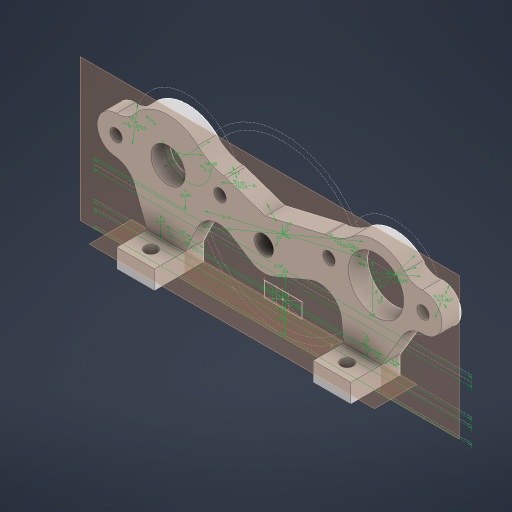
# Autodesk Inventor part: Motormount
Saved by Autodesk Inventor 2023.5 (Build 275446000, 446)
## iProperties
Created: 2024-12-07
Part Number: Motormount
Material: 一般
Document SubType Name: Modeling
Designer: IshiiLabHonda
Density: 1 g/cm^3
Appearance: 既定
Author: IshiiLabHonda
Autodesk Inventor part; units mm, degrees
ref_plane "YZ Plane" through (0, 0, 0) normal (1, 0, 0) x (0, 1, 0)
ref_plane "XZ Plane" through (0, 0, 0) normal (0, 1, 0) x (-1, 0, 0)
ref_plane "XY Plane" through (0, 0, 0) normal (0, 0, 1) x (1, 0, 0)
sketch "blueprint" plane through (0, 0, 0) normal (0, 0, 1) x (1, 0, 0)
  line L0 (0, 0) -> (0, 1) construction
  line L1 (0, 0) -> (1, 0) construction
  circle A0 centre (0, 0) radius 1.25
  circle A1 centre (0, 0) radius 11.5 construction
  line L2 (-25, -11.5) -> (25, -11.5) construction
  line L3 (-25, -9.5) -> (25, -9.5) construction
  line L4 (-25, -8.5) -> (25, -8.5) construction
  line L5 (-25, -4.5) -> (25, -4.5) construction
  circle A2 centre (0, 0) radius 10.65 construction
  circle A3 centre (-12.6949, 2.8) radius 2.25
  circle A4 centre (14.8381, 2.8) radius 4.35 construction
  circle A5 centre (14.8381, 2.8) radius 3.6 construction
  line L6 (-25, -3.7) -> (25, -3.7) construction
  circle A6 centre (-12.6949, 2.8) radius 4.26 construction
  circle A7 centre (-19.5799, 2.8) radius 0.625 construction
  circle A8 centre (-5.8099, 2.8) radius 0.625 construction
  circle A9 centre (-12.6949, 2.8) radius 6.885 construction
  circle A10 centre (-19.5799, 2.8) radius 1.825
  circle A11 centre (-5.8099, 2.8) radius 1.825
  circle A12 centre (14.8381, 2.8) radius 5.1
  circle A13 centre (14.8381, 2.8) radius 6.225 construction
  circle A14 centre (21.0631, 2.8) radius 0.625 construction
  circle A15 centre (8.6131, 2.8) radius 0.625 construction
  circle A16 centre (21.0631, 2.8) radius 1.825
  circle A17 centre (-19.5799, 2.8) radius 0.8
  circle A18 centre (-5.8099, 2.8) radius 0.8
  circle A19 centre (21.0631, 2.8) radius 0.8
  circle A20 centre (-19.5799, 2.8) radius 2.5
  circle A21 centre (-5.8099, 2.8) radius 2.5
  circle A22 centre (21.0631, 2.8) radius 2.5
  circle A23 centre (14.8381, 2.8) radius 3.65
  circle A24 centre (0, 0) radius 3.25
  line L7 (-15, -4.5) -> (-15, -8.5) construction
  line L8 (15, -4.5) -> (15, -8.5) construction
  line L9 (-10.5, -8.5) -> (-10.5, -6)
  line L10 (-15.5, -8.5) -> (-15.5, -6)
  line L11 (-15.5, -6) -> (-10.5, -6)
  line L12 (-13, -6) -> (-13, -8.5)
  line L13 (-13.8, -6) -> (-13.8, -8.5)
  line L14 (-12.2, -6) -> (-12.2, -8.5)
  line L15 (10.5, -8.5) -> (10.5, -6)
  line L16 (15.5, -8.5) -> (15.5, -6)
  line L17 (15.5, -6) -> (10.5, -6)
  line L18 (13, -6) -> (13, -8.5)
  line L19 (13.8, -6) -> (13.8, -8.5)
  line L20 (12.2, -6) -> (12.2, -8.5)
  line L21 (-15.5, -8.5) -> (-10.5, -8.5)
  line L22 (10.5, -8.5) -> (15.5, -8.5)
  circle A25 centre (8.6131, 2.8) radius 1.825
  line L23 (-12.6949, 2.8) -> (-19.5799, 2.8) construction
  line L24 (-12.6949, 2.8) -> (-5.8099, 2.8) construction
  line L25 (14.8381, 2.8) -> (8.6131, 2.8) construction
  circle A26 centre (-12.6949, 2.8) radius 5.76
  line L26 (-2.5, -6.5) -> (2.5, -6.5)
  line L27 (2.5, -6.5) -> (2.5, -8.5)
  line L28 (2.5, -8.5) -> (-2.5, -8.5)
  line L29 (-2.5, -8.5) -> (-2.5, -6.5)
  line L30 (-2.5, -6.5) -> (2.5, -8.5) construction
  line L31 (2.5, -6.5) -> (-2.5, -8.5) construction
  line L32 (0, -6.5) -> (0, -8.5) construction
  line L33 (-0.8, -6.5) -> (-0.8, -8.5) construction
  line L34 (0.8, -6.5) -> (0.8, -8.5) construction
  circle A27 centre (8.6131, 2.8) radius 0.8
  circle A28 centre (8.6131, 2.8) radius 2.5
  line L35 (21.0631, 2.8) -> (14.8381, 2.8) construction
  circle A29 centre (0, 0) radius 2.15
  point P0 (19.5378, 0.8193)
  point P1 (19.5378, 4.7807)
  point P2 (0, -8.5)
  point P3 (-6.4807, -9.5)
  point P4 (6.4807, -9.5)
  point P5 (0, -7.5)
  point P6 (-18.0929, 0.7903)
  point P7 (-7.2969, 0.7903)
  point P8 (-7.2969, 4.8097)
  point P9 (-18.0929, 4.8097)
  dimension "d0" = 1
  dimension "d1" = 1
  dimension "d2" = 2.5
  dimension "d3" = 23
  dimension "d4" = 50
  dimension "d5" = 50
  dimension "d6" = 2
  dimension "d7" = 50
  dimension "d9" = 1
  dimension "d10" = 50
  dimension "d12" = 4
  dimension "d13" = 21.3
  dimension "d14" = 4.5
  dimension "d15" = 8.7
  dimension "d17" = 0.1
  dimension "d18" = 0.1
  dimension "d20" = 7.2
  dimension "d21" = 50
  dimension "d22" = 0.8
  dimension "d23" = 8.52
  dimension "d26" = 1.25
  dimension "d27" = 1.25
  dimension "d28" = 1.2
  dimension "d29" = 1.2
  dimension "d31" = 1.5
  dimension "d32" = 1.25
  dimension "d33" = 1.25
  dimension "d34" = 1.2
  dimension "d37" = 0.5
  dimension "d40" = 1.6
  dimension "d41" = 1.6
  dimension "d43" = 1.6
  dimension "d48" = 7.3
  dimension "d49" = 2
  dimension "d56" = 30
  dimension "d90" = 2.5
  dimension "d92" = 5
  dimension "d93" = 1.6
  dimension "d104" = 1.2
  dimension "d105" = 5
  dimension "d106" = 1.6
  dimension "d107" = 2.5
  dimension "d129" = 5
  dimension "d130" = 5
  dimension "d132" = 5
  dimension "d155" = 26
  dimension "d158" = 1.5
  dimension "d160" = 0.5
  dimension "d161" = 180
  dimension "d166" = 1.6
  dimension "d167" = 5
  dimension "d168" = 2
  dimension "d178" = 1.6
  dimension "d179" = 5
  dimension "d180" = 180
  dimension "d181" = 6.5
  dimension "d187" = 2.24
  dimension "d196" = 4.3
  constraints: 70 end point, 30 centre point, 25 coincident, 17 point on line, 10 parallel, 8 midpoint, 7 vertical, 6 point on circle, 5 symmetric about line, 4 perpendicular, 3 horizontal, 1 tangent, 18 other
  measures "d0" distance of L0.start L0.end
  measures "d1" distance of L0.start L1.end
  measures "d2" diameter of A0
  measures "d3" diameter of A1
  measures "d4" distance of L2.start L2.end
  measures "d5" distance of L3.start L3.end
  measures "d6" distance between parallel lines of L2 L3
  measures "d7" distance of point (-25, -8.5) point (25, -8.5)
  measures "d10" distance of L5.start L5.end
  measures "d13" diameter of A2
  measures "d14" diameter of A3
  measures "d15" diameter of A4
  measures "d20" diameter of A5
  measures "d21" distance of L6.start L6.end
  measures "d22" distance between parallel lines of L5 L6
  measures "d23" diameter of A6
  measures "d26" diameter of A8
  measures "d27" diameter of A7
  measures "d28" radial gap between concentric circles of A10 A7
  measures "d29" radial gap between concentric circles of A11 A8
  measures "d31" radial gap between concentric circles of A12 A5
  measures "d32" diameter of A14
  measures "d33" diameter of A15
  measures "d34" radial gap between concentric circles of A14 A16
  measures "d40" diameter of A17
  measures "d41" diameter of A18
  measures "d43" diameter of A19
  measures "d48" diameter of A23
  measures "d49" radial gap between concentric circles of A24 A0
  measures "d56" distance between parallel lines of L8 L7
  measures "d90" distance of L10.start L10.end
  measures "d92" distance between parallel lines of L9 L10
  measures "d93" distance between parallel lines of L14 L13
  measures "d104" radial gap between concentric circles of A25 A15
  measures "d105" distance between parallel lines of L16 L15
  measures "d106" distance between parallel lines of L19 L20
  measures "d107" distance of L15.start L15.end
  measures "d129" diameter of A20
  measures "d130" diameter of A21
  measures "d132" diameter of A22
  measures "d155" distance between parallel lines of L18 L12
  measures "d158" radial gap between concentric circles of A26 A6
  measures "d161" angle of L24 L23
  measures "d166" distance between parallel lines of L33 L34
  measures "d167" distance between parallel lines of L27 L29
  measures "d168" distance between parallel lines of L26 L28
  measures "d178" diameter of A27
  measures "d179" diameter of A28
  measures "d180" angle of L25 L35
  measures "d181" distance between parallel lines of L6 L25
  measures "d187" distance edge to line of A6 L6
  measures "d196" diameter of A29
sketch "スケッチ5" plane through (0, 0, 0) normal (0, 0, 1) x (1, 0, 0)
  circle A0 centre (0, 0) radius 10.65 construction
  circle A1 centre (0, 0) radius 11.5 construction
  line L0 (-25, -3.7) -> (25, -3.7) construction
  line L1 (-25, -4.5) -> (25, -4.5) construction
  line L2 (-25, -8.5) -> (25, -8.5) construction
  line L3 (-25, -9.5) -> (25, -9.5) construction
  line L4 (-25, -11.5) -> (25, -11.5) construction
  line L5 (0, 0) -> (1, 0) construction
  circle A2 centre (0, 0) radius 1.25 projected
  line L6 (0, 0) -> (0, 1) construction
  circle A3 centre (-5.8099, 2.8) radius 0.625 construction
  circle A4 centre (-5.8099, 2.8) radius 0.8 projected
  circle A5 centre (-5.8099, 2.8) radius 1.825 construction
  circle A6 centre (-5.8099, 2.8) radius 2.5 projected
  line L7 (-12.6949, 2.8) -> (-5.8099, 2.8) construction
  circle A7 centre (-12.6949, 2.8) radius 2.25 projected
  circle A8 centre (-12.6949, 2.8) radius 4.26 construction
  circle A9 centre (-12.6949, 2.8) radius 5.76 projected
  circle A10 centre (-12.6949, 2.8) radius 6.885 construction
  line L8 (-12.6949, 2.8) -> (-19.5799, 2.8) construction
  circle A11 centre (-19.5799, 2.8) radius 2.5 projected
  circle A12 centre (14.8381, 2.8) radius 3.6 construction
  circle A13 centre (14.8381, 2.8) radius 4.35 construction
  circle A14 centre (-19.5799, 2.8) radius 0.625 construction
  circle A15 centre (-19.5799, 2.8) radius 0.8 projected
  circle A16 centre (-19.5799, 2.8) radius 1.825 construction
  circle A17 centre (14.8381, 2.8) radius 5.1 projected
  circle A18 centre (14.8381, 2.8) radius 6.225 construction
  circle A19 centre (21.0631, 2.8) radius 0.625 construction
  circle A20 centre (8.6131, 2.8) radius 0.625 construction
  circle A21 centre (21.0631, 2.8) radius 1.825 construction
  line L9 (14.8381, 2.8) -> (8.6131, 2.8) construction
  circle A22 centre (8.6131, 2.8) radius 0.8 projected
  circle A23 centre (8.6131, 2.8) radius 1.825 construction
  circle A24 centre (8.6131, 2.8) radius 2.5 projected
  circle A25 centre (14.8381, 2.8) radius 3.65 projected
  line L10 (21.0631, 2.8) -> (14.8381, 2.8) construction
  circle A26 centre (21.0631, 2.8) radius 2.5 projected
  circle A27 centre (21.0631, 2.8) radius 0.8 projected
  line L11 (-10.5, -8.5) -> (-10.5, -6) projected
  line L12 (-12.2, -6) -> (-12.2, -8.5) projected
  line L13 (-15.5, -6) -> (-10.5, -6) projected
  line L14 (-13, -6) -> (-13, -8.5) projected
  line L15 (-13.8, -6) -> (-13.8, -8.5) projected
  line L16 (-15.5, -8.5) -> (-10.5, -8.5) projected
  line L17 (-15, -4.5) -> (-15, -8.5) construction
  line L18 (-15.5, -8.5) -> (-15.5, -6) projected
  line L19 (15, -4.5) -> (15, -8.5) construction
  line L20 (15.5, -8.5) -> (15.5, -6) projected
  line L21 (13.8, -6) -> (13.8, -8.5) projected
  line L22 (15.5, -6) -> (10.5, -6) projected
  line L23 (13, -6) -> (13, -8.5) projected
  line L24 (12.2, -6) -> (12.2, -8.5) projected
  line L25 (10.5, -8.5) -> (15.5, -8.5) projected
  line L26 (10.5, -8.5) -> (10.5, -6) projected
  circle A28 centre (0, 0) radius 3.25 projected
  line L27 (-2.5, -8.5) -> (-2.5, -6.5) projected
  line L28 (-0.8, -6.5) -> (-0.8, -8.5) construction
  line L29 (0, -6.5) -> (0, -8.5) construction
  line L30 (0.8, -6.5) -> (0.8, -8.5) construction
  line L31 (-2.5, -6.5) -> (2.5, -6.5) projected
  line L32 (-2.5, -6.5) -> (2.5, -8.5) construction
  line L33 (2.5, -6.5) -> (-2.5, -8.5) construction
  line L34 (2.5, -8.5) -> (-2.5, -8.5) projected
  line L35 (2.5, -6.5) -> (2.5, -8.5) projected
  line L36 (-15.5, -6) -> (-18.0759, 0.7451)
  line L37 (-10.5, -6) -> (-7.4926, 0.3274)
  line L38 (10.5, -6) -> (9.7581, 2.3486)
  line L39 (15.5, -6) -> (19.2096, 0.1731)
  line L40 (-7.1498, 0.6894) -> (-1.7419, -2.7438)
  line L41 (-4.9938, 5.163) -> (1.0609, 3.072)
  line L42 (-0.7454, 3.1634) -> (8.0398, 5.2334)
  line L43 (1.2573, -2.997) -> (9.5803, 0.4946)
  point P0 (0, -7.5)
  point P1 (0, -8.5)
  point P2 (6.4807, -9.5)
  point P3 (-6.4807, -9.5)
  point P4 (10.1385, 0.8193)
  point P5 (9.9081, 0.6615)
  point P6 (0.171, 3.3793)
  point P7 (-18.0929, 4.8097)
  point P8 (-18.0929, 0.7903)
  point P9 (-7.2969, 0.7903)
  point P10 (19.5378, 0.8193)
  point P11 (19.5378, 4.7807)
  point P12 (10.1385, 4.7807)
  point P13 (-7.2969, 4.8097)
  constraints: 16 end point, 12 point on circle, 12 tangent, 5 other
extrude "押し出し33" add sketch "スケッチ5" along normal blind 2.5 contours A6 A9 | A6 L41 L42 A28 L40 | A9 A6 | A6 A9 A11 | L42 A24 L43 A28 L41 | L41 A28 L42 | A28 | A11 A9 | A9 A11 | A24 A17 L38 | L37 L13 L36 A9 | A24 A17 | A17 A26 A24 | L11 L16 L12 L13 | L38 A17 A24 | A24 A17 L39 L22 L38 | A26 A17 | A17 A26 | L13 L15 L16 L18 | L12 L16 L14 L13 | L22 L24 L25 L26 | L13 L14 L16 L15 | L22 L23 L25 L24 | L20 L25 L21 L22 | L22 L21 L25 L23
extrude "押し出し34" cut sketch "blueprint" along normal blind 0.5 contours A10 A26 | A26 A10 | A26 A11 | A11 A26 | A12 A16 | A12 A16 | A25 A12 | A12 A25 | A17 | A19 | A29
fillet "フィレット2" radius 7 2 edges at (10.1385, 4.7807, 1.25) (-7.2969, 4.8097, 1.25)
fillet "フィレット3" radius 3 6 edges at (9.9081, 0.6615, 1.25) (-7.2969, 0.7903, 1.25) (-18.0929, 0.7903, 1.25) (-18.0929, 4.8097, 1.25) (19.5378, 4.7807, 1.25) (19.5378, 0.8193, 1.25)
ref_plane "作業平面6" through (0, 0, 2.5) normal (0, 0, 1) x (1, 0, 0)
sketch "スケッチ7" plane through (0, 0, 2.5) normal (0, 0, 1) x (1, 0, 0)
  line L0 (-4.4189, -1.0443) -> (-1.7419, -2.7438) projected
  line L1 (-10.5, -8.5) -> (-10.5, -6) projected
  line L2 (-10.5, -8.5) -> (-10.5, -6) projected
  line L3 (-4.4189, -1.0443) -> (-1.7419, -2.7438) projected
  line L4 (10.5, -6) -> (10.5, -8.5) projected
  line L5 (10.5, -6) -> (10.5, -8.5) projected
  arc A0 (21.0269, 0.3003) -> (20.9393, 5.2969) centre (21.0631, 2.8) ccw projected
  arc A1 (21.0269, 0.3003) -> (20.9393, 5.2969) centre (21.0631, 2.8) ccw projected
  line L6 (10.5, -8.5) -> (15.5, -8.5) projected
  line L7 (15.5, -8.5) -> (15.5, -6) projected
  line L8 (15.5, -8.5) -> (15.5, -6) projected
  line L9 (10.5, -8.5) -> (15.5, -8.5) projected
  line L10 (-15.5, -6) -> (-15.5, -8.5) projected
  line L11 (-15.5, -6) -> (-15.5, -8.5) projected
  line L12 (-15.5, -8.5) -> (-10.5, -8.5) projected
  line L13 (-15.5, -8.5) -> (-10.5, -8.5) projected
  arc A2 (-4.4189, -1.0443) -> (-8.7363, -2.2892) centre (-6.0267, -3.577) ccw projected
  arc A3 (-1.7419, -2.7438) -> (1.2573, -2.997) centre (0, 0) ccw projected
  arc A4 (-1.7419, -2.7438) -> (1.2573, -2.997) centre (0, 0) ccw projected
  circle A5 centre (-5.8099, 2.8) radius 0.8 projected
  circle A6 centre (-5.8099, 2.8) radius 0.8 projected
  circle A7 centre (0, 0) radius 1.25 projected
  circle A8 centre (-5.8099, 2.8) radius 1.825 projected
  circle A9 centre (-5.8099, 2.8) radius 1.825 projected
  arc A10 (-4.9938, 5.163) -> (-5.329, 5.2533) centre (-5.8099, 2.8) ccw projected
  circle A11 centre (0, 0) radius 2.15 projected
  circle A12 centre (0, 0) radius 2.15 projected
  line L14 (0.171, 3.3793) -> (-4.9938, 5.163) projected
  line L15 (0.171, 3.3793) -> (-4.9938, 5.163) projected
  arc A13 (-8.762, 7.0083) -> (-5.329, 5.2533) centre (-3.9824, 12.1226) ccw projected
  arc A14 (-8.762, 7.0083) -> (-5.329, 5.2533) centre (-3.9824, 12.1226) ccw projected
  line L16 (10.2739, -3.4557) -> (10.5, -6) projected
  line L17 (10.2739, -3.4557) -> (10.5, -6) projected
  line L18 (8.0398, 5.2334) -> (0.171, 3.3793) projected
  line L19 (8.0398, 5.2334) -> (0.171, 3.3793) projected
  arc A15 (8.2451, 5.2728) -> (8.0398, 5.2334) centre (8.6131, 2.8) ccw projected
  arc A16 (8.2451, 5.2728) -> (8.0398, 5.2334) centre (8.6131, 2.8) ccw projected
  circle A17 centre (8.6131, 2.8) radius 0.8 projected
  circle A18 centre (8.6131, 2.8) radius 0.8 projected
  circle A19 centre (8.6131, 2.8) radius 1.825 projected
  circle A20 centre (8.6131, 2.8) radius 1.825 projected
  circle A21 centre (14.8381, 2.8) radius 3.65 projected
  circle A22 centre (14.8381, 2.8) radius 3.65 projected
  circle A23 centre (21.0631, 2.8) radius 0.8 projected
  circle A24 centre (0, 0) radius 1.25 projected
  arc A25 (8.2451, 5.2728) -> (11.625, 6.7605) centre (7.2148, 12.1965) ccw projected
  circle A26 centre (-12.6949, 2.8) radius 2.25 projected
  circle A27 centre (-12.6949, 2.8) radius 2.25 projected
  circle A28 centre (-19.5799, 2.8) radius 0.8 projected
  arc A29 (-8.762, 7.0083) -> (-17.1783, 6.4162) centre (-12.6949, 2.8) ccw projected
  arc A30 (-8.762, 7.0083) -> (-17.1783, 6.4162) centre (-12.6949, 2.8) ccw projected
  line L20 (-17.1744, -1.6154) -> (-15.5, -6) projected
  circle A31 centre (-19.5799, 2.8) radius 0.8 projected
  circle A32 centre (-19.5799, 2.8) radius 1.825 projected
  circle A33 centre (-19.5799, 2.8) radius 1.825 projected
  circle A34 centre (21.0631, 2.8) radius 0.8 projected
  circle A35 centre (21.0631, 2.8) radius 1.825 projected
  circle A36 centre (21.0631, 2.8) radius 1.825 projected
  arc A37 (-4.9938, 5.163) -> (-5.329, 5.2533) centre (-5.8099, 2.8) ccw projected
  line L21 (-17.1744, -1.6154) -> (-15.5, -6) projected
  arc A38 (-4.4189, -1.0443) -> (-8.7363, -2.2892) centre (-6.0267, -3.577) ccw projected
  line L22 (-10.5, -6) -> (-8.7363, -2.2892) projected
  line L23 (-10.5, -6) -> (-8.7363, -2.2892) projected
  arc A39 (8.2451, 5.2728) -> (11.625, 6.7605) centre (7.2148, 12.1965) ccw projected
  line L24 (1.2573, -2.997) -> (6.1251, -0.9548) projected
  line L25 (1.2573, -2.997) -> (6.1251, -0.9548) projected
  arc A40 (10.2739, -3.4557) -> (6.1251, -0.9548) centre (7.2857, -3.7213) ccw projected
  arc A41 (18.5861, 6.2587) -> (11.625, 6.7605) centre (14.8381, 2.8) ccw projected
  arc A42 (18.5861, 6.2587) -> (11.625, 6.7605) centre (14.8381, 2.8) ccw projected
  line L26 (15.5, -6) -> (18.412, -1.1542) projected
  line L27 (15.5, -6) -> (18.412, -1.1542) projected
  arc A43 (10.2739, -3.4557) -> (6.1251, -0.9548) centre (7.2857, -3.7213) ccw projected
  arc A44 (-17.1744, -1.6154) -> (-19.7604, 0.3065) centre (-19.977, -2.6856) ccw projected
  arc A45 (-17.1744, -1.6154) -> (-19.7604, 0.3065) centre (-19.977, -2.6856) ccw projected
  arc A46 (-19.5497, 5.2998) -> (-19.7604, 0.3065) centre (-19.5799, 2.8) ccw projected
  arc A47 (-19.5497, 5.2998) -> (-17.1783, 6.4162) centre (-19.5134, 8.2996) ccw projected
  arc A48 (-19.5497, 5.2998) -> (-19.7604, 0.3065) centre (-19.5799, 2.8) ccw projected
  arc A49 (-19.5497, 5.2998) -> (-17.1783, 6.4162) centre (-19.5134, 8.2996) ccw projected
  arc A50 (21.0269, 0.3003) -> (18.412, -1.1542) centre (20.9834, -2.6994) ccw projected
  arc A51 (21.0269, 0.3003) -> (18.412, -1.1542) centre (20.9834, -2.6994) ccw projected
  arc A52 (18.5861, 6.2587) -> (20.9393, 5.2969) centre (20.7908, 8.2933) ccw projected
  arc A53 (18.5861, 6.2587) -> (20.9393, 5.2969) centre (20.7908, 8.2933) ccw projected
  line L28 (-25, -3.7) -> (25, -3.7) construction
  line L29 (-25, -4.5) -> (25, -4.5) construction
  line L30 (-25, -8.5) -> (25, -8.5) construction
  line L31 (-25, -9.5) -> (25, -9.5) construction
  line L32 (-25, -11.5) -> (25, -11.5) construction
  circle A54 centre (0, 0) radius 10.65 construction
  circle A55 centre (0, 0) radius 11.5 construction
  circle A56 centre (0, 0) radius 1.25 projected
  circle A57 centre (-5.8099, 2.8) radius 0.8 projected
  circle A58 centre (-5.8099, 2.8) radius 1.825 projected
  circle A59 centre (-5.8099, 2.8) radius 2.5 projected
  circle A60 centre (-5.8099, 2.8) radius 0.625 construction
  line L33 (0, 0) -> (0, 1) construction
  circle A61 centre (-12.6949, 2.8) radius 4.26 construction
  line L34 (-12.6949, 2.8) -> (-5.8099, 2.8) construction
  circle A62 centre (-12.6949, 2.8) radius 5.76 projected
  circle A63 centre (-12.6949, 2.8) radius 6.885 construction
  line L35 (0, 0) -> (1, 0) construction
  circle A64 centre (-19.5799, 2.8) radius 0.8 projected
  circle A65 centre (-19.5799, 2.8) radius 1.825 projected
  circle A66 centre (-19.5799, 2.8) radius 2.5 projected
  circle A67 centre (14.8381, 2.8) radius 3.6 construction
  circle A68 centre (14.8381, 2.8) radius 4.35 construction
  line L36 (-12.6949, 2.8) -> (-19.5799, 2.8) construction
  circle A69 centre (-12.6949, 2.8) radius 2.25 projected
  circle A70 centre (-19.5799, 2.8) radius 0.625 construction
  circle A71 centre (14.8381, 2.8) radius 5.1 projected
  circle A72 centre (14.8381, 2.8) radius 6.225 construction
  circle A73 centre (21.0631, 2.8) radius 0.625 construction
  circle A74 centre (8.6131, 2.8) radius 0.625 construction
  line L37 (21.0631, 2.8) -> (14.8381, 2.8) construction
  circle A75 centre (21.0631, 2.8) radius 0.8 projected
  circle A76 centre (21.0631, 2.8) radius 1.825 projected
  circle A77 centre (21.0631, 2.8) radius 2.5 projected
  circle A78 centre (14.8381, 2.8) radius 3.65 projected
  circle A79 centre (8.6131, 2.8) radius 0.8 projected
  circle A80 centre (8.6131, 2.8) radius 1.825 projected
  circle A81 centre (8.6131, 2.8) radius 2.5 projected
  line L38 (14.8381, 2.8) -> (8.6131, 2.8) construction
  line L39 (15.5, -6) -> (10.5, -6) projected
  line L40 (10.5, -8.5) -> (15.5, -8.5) projected
  line L41 (15, -4.5) -> (15, -8.5) construction
  line L42 (12.2, -6) -> (12.2, -8.5) projected
  line L43 (13, -6) -> (13, -8.5) projected
  line L44 (15.5, -8.5) -> (15.5, -6) projected
  line L45 (13.8, -6) -> (13.8, -8.5) projected
  line L46 (10.5, -8.5) -> (10.5, -6) projected
  circle A82 centre (0, 0) radius 3.25 projected
  line L47 (2.5, -6.5) -> (2.5, -8.5) projected
  line L48 (0.8, -6.5) -> (0.8, -8.5) construction
  circle A83 centre (0, 0) radius 2.15 projected
  line L49 (0, -6.5) -> (0, -8.5) construction
  line L50 (-0.8, -6.5) -> (-0.8, -8.5) construction
  line L51 (-2.5, -6.5) -> (2.5, -6.5) projected
  line L52 (-2.5, -6.5) -> (2.5, -8.5) construction
  line L53 (2.5, -8.5) -> (-2.5, -8.5) projected
  line L54 (2.5, -6.5) -> (-2.5, -8.5) construction
  line L55 (-2.5, -8.5) -> (-2.5, -6.5) projected
  line L56 (-15.5, -6) -> (-10.5, -6) projected
  line L57 (-15, -4.5) -> (-15, -8.5) construction
  line L58 (-13, -6) -> (-13, -8.5) projected
  line L59 (-13.8, -6) -> (-13.8, -8.5) projected
  line L60 (-15.5, -8.5) -> (-15.5, -6) projected
  line L61 (-12.2, -6) -> (-12.2, -8.5) projected
  line L62 (-15.5, -8.5) -> (-10.5, -8.5) projected
  line L63 (-10.5, -8.5) -> (-10.5, -6) projected
  line L64 (12.2, -6) -> (12.2, -8.5) projected
  line L65 (13.8, -6) -> (13.8, -8.5) projected
  line L66 (10.5, -8.5) -> (10.5, -6) projected
  line L67 (15.5, -8.5) -> (15.5, -6) projected
  line L68 (15, -4.5) -> (15, -8.5) construction
  line L69 (15.5, -6) -> (10.5, -6) projected
  circle A84 centre (0, 0) radius 10.65 construction
  circle A85 centre (0, 0) radius 11.5 construction
  line L70 (10.5, -6) -> (9.7581, 2.3486) projected
  line L71 (14.8381, 2.8) -> (8.6131, 2.8) construction
  circle A86 centre (8.6131, 2.8) radius 0.625 construction
  circle A87 centre (8.6131, 2.8) radius 0.8 projected
  circle A88 centre (8.6131, 2.8) radius 1.825 construction
  circle A89 centre (8.6131, 2.8) radius 2.5 projected
  line L72 (1.2573, -2.997) -> (9.5803, 0.4946) projected
  line L73 (-25, -11.5) -> (25, -11.5) construction
  line L74 (-25, -9.5) -> (25, -9.5) construction
  line L75 (-25, -8.5) -> (25, -8.5) construction
  line L76 (-25, -3.7) -> (25, -3.7) construction
  line L77 (-25, -4.5) -> (25, -4.5) construction
  line L78 (-0.7454, 3.1634) -> (8.0398, 5.2334) projected
  line L79 (13, -6) -> (13, -8.5) projected
  line L80 (-10.5, -6) -> (-7.4926, 0.3274) projected
  line L81 (-15.5, -6) -> (-18.0759, 0.7451) projected
  line L82 (-12.6949, 2.8) -> (-5.8099, 2.8) construction
  line L83 (-12.6949, 2.8) -> (-19.5799, 2.8) construction
  circle A90 centre (-19.5799, 2.8) radius 0.625 construction
  circle A91 centre (-19.5799, 2.8) radius 0.8 projected
  circle A92 centre (-19.5799, 2.8) radius 1.825 construction
  circle A93 centre (-19.5799, 2.8) radius 2.5 projected
  circle A94 centre (-12.6949, 2.8) radius 6.885 construction
  circle A95 centre (-12.6949, 2.8) radius 5.76 projected
  circle A96 centre (-12.6949, 2.8) radius 4.26 construction
  circle A97 centre (-12.6949, 2.8) radius 2.25 projected
  circle A98 centre (14.8381, 2.8) radius 3.6 construction
  circle A99 centre (14.8381, 2.8) radius 4.35 construction
  circle A100 centre (14.8381, 2.8) radius 5.1 projected
  circle A101 centre (14.8381, 2.8) radius 6.225 construction
  circle A102 centre (21.0631, 2.8) radius 0.625 construction
  circle A103 centre (21.0631, 2.8) radius 1.825 construction
  line L84 (15.5, -6) -> (19.2096, 0.1731) projected
  circle A104 centre (14.8381, 2.8) radius 3.65 projected
  line L85 (21.0631, 2.8) -> (14.8381, 2.8) construction
  circle A105 centre (21.0631, 2.8) radius 0.8 projected
  circle A106 centre (21.0631, 2.8) radius 2.5 projected
  line L86 (-15.5, -6) -> (-10.5, -6) projected
  line L87 (-15, -4.5) -> (-15, -8.5) construction
  line L88 (-15.5, -8.5) -> (-10.5, -8.5) projected
  line L89 (-15.5, -8.5) -> (-15.5, -6) projected
  line L90 (-13.8, -6) -> (-13.8, -8.5) projected
  line L91 (-13, -6) -> (-13, -8.5) projected
  line L92 (-12.2, -6) -> (-12.2, -8.5) projected
  line L93 (-10.5, -8.5) -> (-10.5, -6) projected
  line L94 (0, 0) -> (1, 0) construction
  circle A107 centre (0, 0) radius 1.25 projected
  line L95 (0, 0) -> (0, 1) construction
  circle A108 centre (-5.8099, 2.8) radius 0.625 construction
  circle A109 centre (-5.8099, 2.8) radius 0.8 projected
  circle A110 centre (-5.8099, 2.8) radius 1.825 construction
  circle A111 centre (-5.8099, 2.8) radius 2.5 projected
  line L96 (-7.1498, 0.6894) -> (-1.7419, -2.7438) projected
  line L97 (-2.5, -8.5) -> (-2.5, -6.5) projected
  line L98 (-0.8, -6.5) -> (-0.8, -8.5) construction
  line L99 (0, -6.5) -> (0, -8.5) construction
  line L100 (-4.9938, 5.163) -> (1.0609, 3.072) projected
  circle A112 centre (0, 0) radius 3.25 projected
  line L101 (0.8, -6.5) -> (0.8, -8.5) construction
  line L102 (2.5, -6.5) -> (2.5, -8.5) projected
  line L103 (-2.5, -6.5) -> (2.5, -8.5) construction
  line L104 (2.5, -6.5) -> (-2.5, -8.5) construction
  line L105 (2.5, -8.5) -> (-2.5, -8.5) projected
  line L106 (-2.5, -6.5) -> (2.5, -6.5) projected
  line L107 (10.5, -8.5) -> (15.5, -8.5) projected
  point P0 (0, -7.5)
  point P1 (0, -8.5)
  point P2 (6.4807, -9.5)
  point P3 (-6.4807, -9.5)
  point P4 (-6.4807, -9.5)
  point P5 (6.4807, -9.5)
  point P6 (0, -8.5)
  point P7 (0, -7.5)
  constraints: 26 other
extrude "押し出し37" add sketch "スケッチ7" along normal blind 4 contours L1 L12 L61 L56 | L61 L12 L58 L56 | L58 L12 L59 L56 | L39 L42 L6 L4 | L59 L12 L10 L56 | L39 L43 L6 L42 | L39 L45 L6 L43 | L39 L7 L6 L45
ref_plane "作業平面7" through (-15.5, -6, 2.5) normal (0, 1, 0) x (1, 0, 0)
sketch "スケッチ8" plane through (-15.5, -6, 2.5) normal (0, 1, 0) x (1, 0, 0)
  line L0 (26, 2.5) -> (26, 0) projected
  line L1 (24.9131, 0) -> (23.3131, 0) projected
  line L2 (21.6251, 0) -> (25.7739, 0) projected
  line L3 (25.7739, 0) -> (26, 0) projected
  line L4 (31, 2.5) -> (31, 0) projected
  line L5 (26, 2.5) -> (31, 2.5) projected
  line L6 (37.3631, 0) -> (35.7631, 0) projected
  line L7 (0, 2.5) -> (0, 0) projected
  line L8 (5, 2.5) -> (5, 0) projected
  line L9 (0, 2.5) -> (5, 2.5) projected
  line L10 (16.75, 0) -> (14.25, 0) projected
  line L11 (10.171, 0) -> (10.5062, 0) projected
  line L12 (10.4901, 0) -> (8.8901, 0) projected
  line L13 (6.7637, 0) -> (11.0811, 0) projected
  line L14 (5, 0) -> (6.7637, 0) projected
  line L15 (5.0551, 0) -> (0.5551, 0) projected
  line L16 (-1.6744, 0) -> (0, 0) projected
  line L17 (-4.2604, 0) -> (-1.6744, 0) projected
  line L18 (-4.0497, 0) -> (-1.6783, 0) projected
  line L19 (-3.2799, 0) -> (-4.8799, 0) projected
  line L20 (-6.5799, 0) -> (-4.0497, 0) projected
  line L21 (23.5398, 0) -> (23.7451, 0) projected
  line L22 (31, 0) -> (33.912, 0) projected
  line L23 (33.912, 0) -> (36.5269, 0) projected
  line L24 (36.4393, 0) -> (39.0631, 0) projected
  line L25 (0, 2.5) -> (0, -4) projected
  line L26 (5, 2.5) -> (5, -4) projected
  line L27 (5, 0) -> (5, -4) projected
  line L28 (5, -4) -> (0, -4) projected
  line L29 (0, 0) -> (0, -4) projected
  line L30 (0, 0) -> (5, 0) projected
  line L31 (31, 0) -> (31, -4) projected
  line L32 (31, -4) -> (26, -4) projected
  line L33 (26, -4) -> (31, -4) projected
  line L34 (0, -4) -> (5, -4) projected
  line L35 (11.0811, 0) -> (13.7581, 0) projected
  line L36 (13.7581, 0) -> (16.7573, 0) projected
  line L37 (13.7581, 2.5) -> (16.7573, 2.5) projected
  line L38 (16.7573, 0) -> (21.6251, 0) projected
  line L39 (23.5398, 0) -> (15.671, 0) projected
  line L40 (15.671, 0) -> (10.5062, 0) projected
  line L41 (13.7581, 2.5) -> (13.7581, 0) projected
  line L42 (26, 2.5) -> (26, -4) projected
  line L43 (31, 2.5) -> (31, -4) projected
  line L44 (25.7739, 2.5) -> (26, 2.5) projected
  line L45 (26, 0) -> (26, -4) projected
  line L46 (26, 0) -> (31, 0) projected
  line L47 (-1.6744, 2.5) -> (0, 2.5) projected
  line L48 (6.7637, 0) -> (6.7637, 2.5) projected
  line L49 (5, 2.5) -> (6.7637, 2.5) projected
  line L50 (16.7573, 2.5) -> (16.7573, 0) projected
  line L51 (25.7739, 2.5) -> (25.7739, 0) projected
  line L52 (-1.6744, 2.5) -> (-1.6744, 0) projected
  line L53 (31, 2.5) -> (26, 2.5) projected
  line L54 (26, 2.5) -> (31, 2.5) projected
  line L55 (13, 2.5) -> (18, 2.5) projected
  line L56 (13, 2.5) -> (18, 2.5) construction
  line L57 (18, 2.5) -> (13, 2.5) projected
  line L58 (18, 2.5) -> (13, 2.5) construction
  line L59 (0, 2.5) -> (5, 2.5) projected
  line L60 (0, 2.5) -> (5, 2.5) projected
  line L61 (31, 2.5) -> (26, 2.5) projected
  line L62 (0, 2.5) -> (5, 2.5) projected
  line L63 (0, 2.5) -> (5, 2.5) projected
  line L64 (13, 2.5) -> (18, 2.5) construction
  line L65 (18, 2.5) -> (13, 2.5) construction
  line L66 (18, 2.5) -> (13, 2.5) projected
  line L67 (13, 2.5) -> (18, 2.5) projected
  line L68 (26, 2.5) -> (31, 2.5) projected
  line L69 (33.9881, 0) -> (26.6881, 0) projected
  line L70 (10.171, 2.5) -> (10.5062, 2.5) projected
  line L71 (10.4901, 2) -> (8.8901, 2) projected
  line L72 (7.8651, 2) -> (11.5151, 2) projected
  line L73 (7.8651, 2.5) -> (11.5151, 2.5) projected
  line L74 (6.7637, 2.5) -> (11.0811, 2.5) projected
  line L75 (10.171, 2.5) -> (6.738, 2.5) projected
  line L76 (6.738, 0) -> (10.171, 0) projected
  line L77 (-1.6783, 0) -> (6.738, 0) projected
  line L78 (23.7451, 0) -> (27.125, 0) projected
  line L79 (27.125, 0) -> (34.0861, 0) projected
  line L80 (34.0861, 0) -> (36.4393, 0) projected
  line L81 (10.5062, 2.5) -> (10.5062, 0) projected
  line L82 (15.671, 2.5) -> (15.671, 0) projected
  line L83 (15.671, 2.5) -> (10.5062, 2.5) projected
  line L84 (13.35, 2) -> (17.65, 2) projected
  line L85 (13.35, 2.5) -> (17.65, 2.5) projected
  line L86 (23.5398, 2.5) -> (15.671, 2.5) projected
  line L87 (11.0811, 2.5) -> (13.7581, 2.5) projected
  line L88 (36.4393, 2.5) -> (39.0631, 2.5) projected
  line L89 (23.5398, 2.5) -> (23.7451, 2.5) projected
  line L90 (24.9131, 2) -> (23.3131, 2) projected
  line L91 (22.2881, 2) -> (25.9381, 2) projected
  line L92 (22.2881, 2.5) -> (25.9381, 2.5) projected
  line L93 (33.9881, 2.5) -> (26.6881, 2.5) projected
  line L94 (23.5398, 2.5) -> (23.5398, 0) projected
  line L95 (16.75, 2) -> (14.25, 2) projected
  line L96 (5.0551, 2.5) -> (0.5551, 2.5) projected
  line L97 (6.738, 2.5) -> (6.738, 0) projected
  line L98 (-1.6783, 2.5) -> (6.738, 2.5) projected
  line L99 (-3.2799, 2) -> (-4.8799, 2) projected
  line L100 (-5.9049, 2.5) -> (-2.2549, 2.5) projected
  line L101 (-5.9049, 2) -> (-2.2549, 2) projected
  line L102 (37.3631, 2) -> (35.7631, 2) projected
  line L103 (34.7381, 2.5) -> (38.3881, 2.5) projected
  line L104 (34.7381, 2) -> (38.3881, 2) projected
  line L105 (10.171, 0) -> (10.171, 2.5) projected
  line L106 (23.7451, 2.5) -> (23.7451, 0) projected
  line L107 (27.125, 2.5) -> (23.7451, 2.5) projected
  line L108 (16.7573, 2.5) -> (21.6251, 2.5) projected
  line L109 (21.6251, 0) -> (21.6251, 2.5) projected
  line L110 (27.125, 2.5) -> (34.0861, 2.5) projected
  line L111 (31, 2.5) -> (33.912, 2.5) projected
  line L112 (27.125, 0) -> (27.125, 2.5) projected
  line L113 (21.6251, 2.5) -> (25.7739, 2.5) projected
  line L114 (-4.2604, 2.5) -> (-1.6744, 2.5) projected
  line L115 (-4.2604, 0) -> (-4.2604, 2.5) projected
  line L116 (-1.6783, 0) -> (-1.6783, 2.5) projected
  line L117 (-4.0497, 2.5) -> (-4.0497, 0) projected
  line L118 (-1.6783, 2.5) -> (-4.0497, 2.5) projected
  line L119 (-6.5799, 2.5) -> (-4.0497, 2.5) projected
  line L120 (33.912, 0) -> (33.912, 2.5) projected
  line L121 (33.912, 2.5) -> (36.5269, 2.5) projected
  line L122 (36.5269, 2.5) -> (36.5269, 0) projected
  line L123 (34.0861, 2.5) -> (34.0861, 0) projected
  line L124 (36.4393, 0) -> (36.4393, 2.5) projected
  line L125 (36.4393, 2.5) -> (34.0861, 2.5) projected
  line L126 (11.0811, 2.5) -> (11.0811, 0) projected
  line L127 (50.5, 0) -> (-19.5, 0) projected
  line L128 (-9.5, 2.5) -> (40.5, 2.5) construction
  line L129 (-9.5, 2.5) -> (40.5, 2.5) construction
  line L130 (-9.5, 2.5) -> (40.5, 2.5) construction
  line L131 (-9.5, 2.5) -> (40.5, 2.5) construction
  line L132 (-9.5, 2.5) -> (40.5, 2.5) construction
  line L133 (4.85, 2.5) -> (26.15, 2.5) construction
  line L134 (4, 2.5) -> (27, 2.5) construction
  line L135 (14.25, 2.5) -> (16.75, 2.5) projected
  line L136 (8.8901, 2.5) -> (10.4901, 2.5) projected
  line L137 (7.8651, 2.5) -> (11.5151, 2.5) projected
  line L138 (7.1901, 2.5) -> (12.1901, 2.5) projected
  line L139 (9.0651, 2.5) -> (10.3151, 2.5) construction
  line L140 (-1.4549, 2.5) -> (7.0651, 2.5) construction
  line L141 (2.8051, 2.5) -> (9.6901, 2.5) construction
  line L142 (-2.9549, 2.5) -> (8.5651, 2.5) projected
  line L143 (-4.0799, 2.5) -> (9.6901, 2.5) construction
  line L144 (15.5, 2.5) -> (16.5, 2.5) construction
  line L145 (-4.8799, 2.5) -> (-3.2799, 2.5) projected
  line L146 (-5.9049, 2.5) -> (-2.2549, 2.5) projected
  line L147 (-6.5799, 2.5) -> (-1.5799, 2.5) projected
  line L148 (26.7381, 2.5) -> (33.9381, 2.5) construction
  line L149 (25.9881, 2.5) -> (34.6881, 2.5) construction
  line L150 (2.8051, 2.5) -> (-4.0799, 2.5) construction
  line L151 (0.5551, 2.5) -> (5.0551, 2.5) projected
  line L152 (-4.7049, 2.5) -> (-3.4549, 2.5) construction
  line L153 (25.2381, 2.5) -> (35.4381, 2.5) projected
  line L154 (24.1131, 2.5) -> (36.5631, 2.5) construction
  line L155 (35.9381, 2.5) -> (37.1881, 2.5) construction
  line L156 (23.4881, 2.5) -> (24.7381, 2.5) construction
  line L157 (36.5631, 2.5) -> (30.3381, 2.5) construction
  line L158 (35.7631, 2.5) -> (37.3631, 2.5) projected
  line L159 (34.7381, 2.5) -> (38.3881, 2.5) projected
  line L160 (34.0631, 2.5) -> (39.0631, 2.5) projected
  line L161 (26.6881, 2.5) -> (33.9881, 2.5) projected
  line L162 (23.3131, 2.5) -> (24.9131, 2.5) projected
  line L163 (22.2881, 2.5) -> (25.9381, 2.5) projected
  line L164 (21.6131, 2.5) -> (26.6131, 2.5) projected
  line L165 (30.3381, 2.5) -> (24.1131, 2.5) construction
  line L166 (12.25, 2.5) -> (18.75, 2.5) projected
  line L167 (13.35, 2.5) -> (17.65, 2.5) projected
  line L168 (4.85, 2.5) -> (26.15, 2.5) construction
  line L169 (4, 2.5) -> (27, 2.5) construction
  line L170 (26, 2.5) -> (25.2581, 2.5) projected
  line L171 (30.3381, 2.5) -> (24.1131, 2.5) construction
  line L172 (23.4881, 2.5) -> (24.7381, 2.5) construction
  line L173 (23.3131, 2.5) -> (24.9131, 2.5) projected
  line L174 (22.2881, 2.5) -> (25.9381, 2.5) construction
  line L175 (21.6131, 2.5) -> (26.6131, 2.5) projected
  line L176 (16.7573, 2.5) -> (25.0803, 2.5) projected
  line L177 (-9.5, 2.5) -> (40.5, 2.5) construction
  line L178 (-9.5, 2.5) -> (40.5, 2.5) construction
  line L179 (-9.5, 2.5) -> (40.5, 2.5) construction
  line L180 (-9.5, 2.5) -> (40.5, 2.5) construction
  line L181 (-9.5, 2.5) -> (40.5, 2.5) construction
  line L182 (14.7546, 2.5) -> (23.5398, 2.5) projected
  line L183 (5, 2.5) -> (8.0074, 2.5) projected
  line L184 (0, 2.5) -> (-2.5759, 2.5) projected
  line L185 (2.8051, 2.5) -> (9.6901, 2.5) construction
  line L186 (2.8051, 2.5) -> (-4.0799, 2.5) construction
  line L187 (-4.7049, 2.5) -> (-3.4549, 2.5) construction
  line L188 (-4.8799, 2.5) -> (-3.2799, 2.5) projected
  line L189 (-5.9049, 2.5) -> (-2.2549, 2.5) construction
  line L190 (-6.5799, 2.5) -> (-1.5799, 2.5) projected
  line L191 (-4.0799, 2.5) -> (9.6901, 2.5) construction
  line L192 (-2.9549, 2.5) -> (8.5651, 2.5) projected
  line L193 (-1.4549, 2.5) -> (7.0651, 2.5) construction
  line L194 (0.5551, 2.5) -> (5.0551, 2.5) projected
  line L195 (26.7381, 2.5) -> (33.9381, 2.5) construction
  line L196 (25.9881, 2.5) -> (34.6881, 2.5) construction
  line L197 (25.2381, 2.5) -> (35.4381, 2.5) projected
  line L198 (24.1131, 2.5) -> (36.5631, 2.5) construction
  line L199 (35.9381, 2.5) -> (37.1881, 2.5) construction
  line L200 (34.7381, 2.5) -> (38.3881, 2.5) construction
  line L201 (31, 2.5) -> (34.7096, 2.5) projected
  line L202 (26.6881, 2.5) -> (33.9881, 2.5) projected
  line L203 (36.5631, 2.5) -> (30.3381, 2.5) construction
  line L204 (35.7631, 2.5) -> (37.3631, 2.5) projected
  line L205 (34.0631, 2.5) -> (39.0631, 2.5) projected
  line L206 (15.5, 2.5) -> (16.5, 2.5) construction
  line L207 (14.25, 2.5) -> (16.75, 2.5) projected
  line L208 (9.0651, 2.5) -> (10.3151, 2.5) construction
  line L209 (8.8901, 2.5) -> (10.4901, 2.5) projected
  line L210 (7.8651, 2.5) -> (11.5151, 2.5) construction
  line L211 (7.1901, 2.5) -> (12.1901, 2.5) projected
  line L212 (8.3502, 2.5) -> (13.7581, 2.5) projected
  line L213 (10.5062, 2.5) -> (16.5609, 2.5) projected
  line L214 (12.25, 2.5) -> (18.75, 2.5) projected
  line L215 (5, -4) -> (0, 0) construction
  line L216 (0, -4) -> (5.0551, 0) construction
  line L217 (26, -4) -> (31, 0) construction
  line L218 (31, -4) -> (26, 0) construction
  circle A0 centre (2.5276, -2) radius 0.8
  circle A1 centre (28.5, -2) radius 0.8
  point P0 (3.3, 2.5)
  point P1 (30.5, 2.5)
  point P2 (27.7, 2.5)
  point P3 (28.5, 2.5)
  point P4 (29.3, 2.5)
  point P5 (30.5, 2.5)
  point P6 (30.5, 2.5)
  point P7 (27.7, 2.5)
  point P8 (27.7, 2.5)
  point P9 (28.5, 2.5)
  point P10 (28.5, 2.5)
  point P11 (29.3, 2.5)
  point P12 (29.3, 2.5)
  point P13 (16.3, 2.5)
  point P14 (16.3, 2.5)
  point P15 (16.3, 2.5)
  point P16 (15.5, 2.5)
  point P17 (14.7, 2.5)
  point P18 (14.7, 2.5)
  point P19 (14.7, 2.5)
  point P20 (0.5, 2.5)
  point P21 (3.3, 2.5)
  point P22 (2.5, 2.5)
  point P23 (0.5, 2.5)
  point P24 (0.5, 2.5)
  point P25 (2.5, 2.5)
  point P26 (2.5, 2.5)
  point P27 (1.7, 2.5)
  point P28 (1.7, 2.5)
  point P29 (1.7, 2.5)
  point P30 (3.3, 2.5)
  point P31 (21.9807, 2.5)
  point P32 (9.0193, 2.5)
  point P33 (27.7, 2.5)
  point P34 (27.7, 2.5)
  point P35 (27.7, 2.5)
  point P36 (29.3, 2.5)
  point P37 (29.3, 2.5)
  point P38 (29.3, 2.5)
  point P39 (30.5, 2.5)
  point P40 (30.5, 2.5)
  point P41 (30.5, 2.5)
  point P42 (28.5, 2.5)
  point P43 (28.5, 2.5)
  point P44 (28.5, 2.5)
  point P45 (0.5, 2.5)
  point P46 (0.5, 2.5)
  point P47 (0.5, 2.5)
  point P48 (1.7, 2.5)
  point P49 (1.7, 2.5)
  point P50 (1.7, 2.5)
  point P51 (2.5, 2.5)
  point P52 (2.5, 2.5)
  point P53 (2.5, 2.5)
  point P54 (3.3, 2.5)
  point P55 (3.3, 2.5)
  point P56 (3.3, 2.5)
  point P57 (14.7, 2.5)
  point P58 (14.7, 2.5)
  point P59 (14.7, 2.5)
  point P60 (16.3, 2.5)
  point P61 (16.3, 2.5)
  point P62 (16.3, 2.5)
  point P63 (9.0193, 2.5)
  point P64 (21.9807, 2.5)
  point P65 (15.5, 2.5)
  dimension "d211" = 1.6
  dimension "d212" = 1.6
  constraints: 8 end point, 8 vertical, 7 horizontal alignment, 4 vertical alignment, 2 centre point, 2 coincident, 2 horizontal, 2 midpoint, 2 perpendicular, 98 other
  measures "d211" diameter of A0
  measures "d212" diameter of A1
extrude "押し出し38" cut sketch "スケッチ8" against normal blind 4 contours A0 | A1
equation "\"d5\" = d4"
equation "\"d7\" = d4"
equation "\"d10\" = d4"
